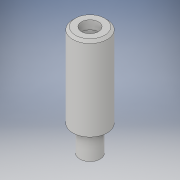
# Autodesk Inventor part: M211L01W-actuator
Saved by Autodesk Inventor 2019 (Build 230136000, 136)
## iProperties
Created: 2022-08-22
Part Number: M211L01W-actuator
Material: Generic
Catalog Web Link: www.cadenas.de
Description: Series M2100 - LED Tipped Actuators -actuator-
Vendor: NKKSWITCHES
Document SubType Name: Modeling
Designer: psAdmin
Manufacturer: NKKSWITCHES
Mass: 0.258535 g
Surface Area: 2.72614 cm^2
Volume: 0.258535 cm^3
Density: 1 g/cm^3
Appearance: PSOLRGB-191-191-191
Category: PARTsolutions
Company: NKKSWITCHES
Title: M211L01W-actuator
Author: Cadenas PARTsolutions
PSOL_IDENT_0: {$CADENAS_DATA/23d-libs/nkkswitches/toggle/m2100/parts/m2100_actuator.prj},230 {VTYP=3D},{NB=M211L01
PSOL_IDENT_1: W-actuator},{LINA=M211L01W-actuator},{NN=Series M2100 - LED Tipped Actuators -actuator},{DATE=02.08.
PSOL_IDENT_2: 2022 07:27:12},{GEOMDATE=23.04.2009 12:14:00},{VERSION=},{LINEID=10},{WBVAR=PLS,LCAT,TMT,CMRT},{WBNU
PSOL_IDENT_3: MERIC=}  {NB=M211L01W-actuator},{LINA=M211L01W-actuator},{KT=DUMMY},{PN=M211L01W},{SRS=M21},{PLS=1},
PSOL_IDENT_4: {LCAT=L},{LCAT1= 'L','L - Isolated (Toggle)','T','T - Synchronous (Toggle)','R','R - Isolated (Rocke
PSOL_IDENT_5: r)','N','N - Synchronous (Rocker)','P','P - Isolated (Paddle)','J','J - Synchronous (Paddle)' },{ACT
PSOL_IDENT_6: UCLR=0.75,0.75,0.75,0.00},{TMT=01},{TMT1= '01','01 - Solder Lug with Threaded Bushing','02','02 - Qu
PSOL_IDENT_7: ick Connect with Threaded Bushing','03','03 - Straight PC with Threaded Bushing' },{CMRT=W}
NB: M211L01W-actuator
NN: Series M2100 - LED Tipped Actuators -actuator
NBSYN: $PN.-actuator
LINA: M211L01W-actuator
CATALOG: NKK Switches
PN: M211L01W
SRS: M21
PLS: 1 - SPDT
LCAT: L - Isolated (Toggle)
TMT: 01 - Solder Lug with Threaded Bushing
CMRT: W - Silver; Rated 6A @ 125V AC
SUPPLIER: NKKSWITCHES
ARTICLENO: M211L01W-actuator
BOMINFO: M211L01W-actuator
CREATOR: CADENAS GmbH
Autodesk Inventor part; units mm, degrees
sketch "Sketch_1" plane through (0, 0, 0) normal (1, 0, 0) x (0, 1, 0)
  line L0 (-1.27, 0) -> (13.4366, 0)
  line L1 (13.4366, 0) -> (13.4366, -1.2446)
  line L2 (13.4366, -1.2446) -> (14.7066, -1.2446)
  line L3 (14.7066, -1.2446) -> (14.7066, -2.1427)
  line L4 (14.7066, -2.1427) -> (14.3474, -2.5019)
  line L5 (14.3474, -2.5019) -> (2.54, -2.5019)
  line L6 (2.54, -2.5019) -> (2.54, -1.4859)
  line L7 (2.54, -1.4859) -> (-1.27, -1.4859)
  line L8 (-1.27, -1.4859) -> (-1.27, 0)
  line L9 (-1.27, 0) -> (13.4366, 0)
  constraints: 20 end point
revolve "Revolution1" add sketch "Sketch_1" angle 360 about axis through (0, -1.27, 0) along (0, -1, 0)
ref_plane "paddle_to_bracket_XY" through (0, -1.3716, 0) normal (0, 0, -1) x (1, 0, 0)
ref_plane "paddle_to_bracket_YZ" through (0, -1.3716, 0) normal (1, 0, 0) x (0, -1, 0)
ref_plane "paddle_to_bracket_ZX" through (0, -1.3716, 0) normal (0, -1, 0) x (0, 0, -1)
ref_plane "paddle_to_led_XY" through (0, 13.8525, 0) normal (0, 1, 0) x (1, 0, 0)
ref_plane "paddle_to_led_YZ" through (0, 13.8525, 0) normal (1, 0, 0) x (0, 0, -1)
ref_plane "paddle_to_led_ZX" through (0, 13.8525, 0) normal (0, 0, -1) x (0, 1, 0)
ref_plane "paddle_to_led_green_XY" through (0, 13.8525, 0) normal (0, 1, 0) x (1, 0, 0)
ref_plane "paddle_to_led_green_YZ" through (0, 13.8525, 0) normal (1, 0, 0) x (0, 0, -1)
ref_plane "paddle_to_led_green_ZX" through (0, 13.8525, 0) normal (0, 0, -1) x (0, 1, 0)
ref_plane "rocker_to_bracket_XY" through (0, 1.778, 0) normal (0, -1, 0) x (1, 0, 0)
ref_plane "rocker_to_bracket_YZ" through (0, 1.778, 0) normal (1, 0, 0) x (0, 0, 1)
ref_plane "rocker_to_bracket_ZX" through (0, 1.778, 0) normal (0, 0, 1) x (0, -1, 0)
ref_plane "toggle_to_bc_XY" through (0, 0, 0) normal (0, 1, 0) x (1, 0, 0)
ref_plane "toggle_to_bc_YZ" through (0, 0, 0) normal (1, 0, 0) x (0, 0, -1)
ref_plane "toggle_to_bc_ZX" through (0, 0, 0) normal (0, 0, -1) x (0, 1, 0)
ref_plane "toggle_to_led_XY" through (0, 13.4366, 0) normal (0, 1, 0) x (1, 0, 0)
ref_plane "toggle_to_led_YZ" through (0, 13.4366, 0) normal (1, 0, 0) x (0, 0, -1)
ref_plane "toggle_to_led_ZX" through (0, 13.4366, 0) normal (0, 0, -1) x (0, 1, 0)
ref_plane "toggle_to_led_green_XY" through (0, 13.4366, 0) normal (0, 1, 0) x (1, 0, 0)
ref_plane "toggle_to_led_green_YZ" through (0, 13.4366, 0) normal (1, 0, 0) x (0, 0, -1)
ref_plane "toggle_to_led_green_ZX" through (0, 13.4366, 0) normal (0, 0, -1) x (0, 1, 0)
body "Solid1"
